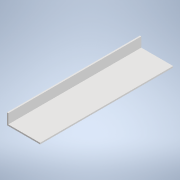
# Autodesk Inventor part: shootingGuide
Saved by Autodesk Inventor 2021 (Build 250183000, 183)
## iProperties
Created: 2020-09-12
Part Number: shootingGuide
Material: Generic
Document SubType Name: Modeling
Designer: deli
Density: 1 g/cm^3
Appearance: Default
Author: deli
Autodesk Inventor part; units mm, degrees
ref_plane "YZ Plane" through (0, 0, 0) normal (1, 0, 0) x (0, 1, 0)
ref_plane "XZ Plane" through (0, 0, 0) normal (0, 1, 0) x (-1, 0, 0)
ref_plane "XY Plane" through (0, 0, 0) normal (0, 0, 1) x (1, 0, 0)
sketch "Sketch1" plane through (0, 0, 0) normal (0, 0, 1) x (1, 0, 0)
  line L0 (-150.6966, 69.1379) -> (-147.5216, 69.1379)
  line L1 (-147.5216, 69.1379) -> (-147.5216, 43.7379)
  line L2 (-147.5216, 43.7379) -> (-150.6966, 43.7379)
  line L3 (-150.6966, 43.7379) -> (-150.6966, 69.1379)
  line L4 (-150.6966, 43.7379) -> (-74.4966, 43.7379)
  line L5 (-74.4966, 43.7379) -> (-74.4966, 46.9129)
  line L6 (-74.4966, 46.9129) -> (-150.6966, 46.9129)
  line L7 (-150.6966, 46.9129) -> (-150.6966, 43.7379)
  point P0 (0, 0)
  point P1 (-147.5216, 46.9129)
  dimension "d0" = 3.175
  dimension "d1" = 25.4
  dimension "d2" = 76.2
  dimension "d3" = 3.175
  constraints: 16 end point, 4 parallel, 2 horizontal, 2 perpendicular
  measures "d0" distance of L1.end L2.end
  measures "d1" distance of L0.end L1.end
  measures "d2" distance of L6.end L5.end
  measures "d3" distance of L5.end L4.end
extrude "Extrusion1" add sketch "Sketch1" along normal blind 304.8
body "Solid1"
